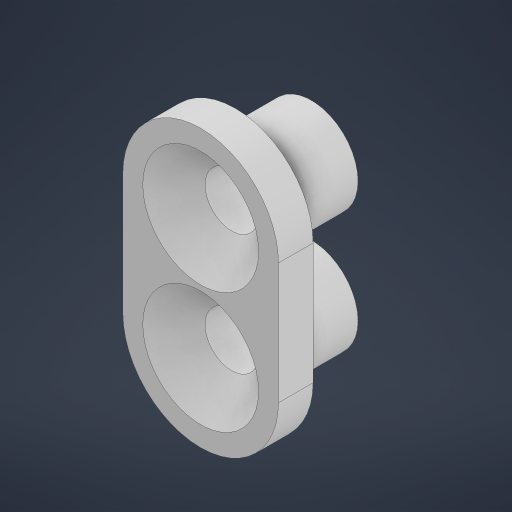
# Autodesk Inventor part: Stange halter
Saved by Autodesk Inventor 2024.2 (Build 282272000, 272)
## iProperties
Created: 2024-02-24
Part Number: Stange halter
Material: Generisch
Document SubType Name: Modeling
Designer: jacob
Density: 1 g/cm^3
Appearance: Vorgabe
Author: jacob
Autodesk Inventor part; units mm, degrees
ref_plane "YZ Plane" through (0, 0, 0) normal (1, 0, 0) x (0, 1, 0)
ref_plane "XZ Plane" through (0, 0, 0) normal (0, 1, 0) x (-1, 0, 0)
ref_plane "XY Plane" through (0, 0, 0) normal (0, 0, 1) x (1, 0, 0)
sketch "Skizze1" plane through (0, 0, 0) normal (0, 0, 1) x (1, 0, 0)
  circle A0 centre (0, 0) radius 2.7
  circle A1 centre (0, -7) radius 2.7
  dimension "d22" = 5.4
  dimension "d23" = 7
  constraints: 2 centre point, 1 coincident, 1 equal radius, 1 vertical alignment
  measures "d22" diameter of A0
  measures "d23" distance of point (0, 0) A1.centre
extrude "Extrusion1" add sketch "Skizze1" along normal blind 5.2
sketch "Skizze2" plane through (0, 0, 5.2) normal (0, 0, 1) x (1, 0, 0)
  arc A0 (-3, -7) -> (3, -7) centre (0, -7) ccw projected
  arc A1 (-3, -7) -> (3, -7) centre (0, -7) ccw projected
  line L0 (-3, 0) -> (-3, -7)
  arc A2 (3, 0) -> (-3, 0) centre (0, 0) ccw
  line L1 (3, -7) -> (3, 0)
  arc A3 (-3, -7) -> (3, -7) centre (0, -7) ccw
  line L2 (-3, 0) -> (-3, -7) projected
  arc A4 (-3, -7) -> (3, -7) centre (0, -7) ccw projected
  line L3 (3, -7) -> (3, 0) projected
  arc A5 (3, 0) -> (-3, 0) centre (0, 0) ccw projected
  line L4 (-3, 0) -> (-3, -7) projected
  line L5 (-3, 0) -> (-3, -7) projected
  arc A6 (-3, -7) -> (3, -7) centre (0, -7) ccw projected
  arc A7 (-3, -7) -> (3, -7) centre (0, -7) ccw projected
  line L6 (3, -7) -> (3, 0) projected
  line L7 (3, -7) -> (3, 0) projected
  arc A8 (3, 0) -> (-3, 0) centre (0, 0) ccw projected
  arc A9 (3, 0) -> (-3, 0) centre (0, 0) ccw projected
  line L8 (-4.5, 0) -> (-4.5, -7)
  arc A10 (-4.5, -7) -> (4.5, -7) centre (0, -7) ccw
  line L9 (4.5, -7) -> (4.5, 0)
  arc A11 (4.5, 0) -> (-4.5, 0) centre (0, 0) ccw
  dimension "d4" = 9
  constraints: 6 end point, 4 centre point, 4 point on circle, 4 tangent, 3 coincident, 1 parallel, 1 vertical
  measures "d4" distance between parallel lines of L8 L9
extrude "Extrusion2" add sketch "Skizze2" along normal blind 2 contours L0 A2 L1 A0 | A11 L9 A10 L8
sketch "Skizze3" plane through (0, 0, 7.2) normal (0, 0, 1) x (1, 0, 0)
  point P0 (0, 0)
  point P1 (0, 0)
  point P2 (0, -7)
  dimension "d7" = 7
  constraints: 1 coincident, 1 vertical alignment
  measures "d7" distance of point (0, 0) point (0, -7)
hole "Bohrung1" at (0, 0, 7.2) at (0, -7, 7.2) direction (0, 0, -1) diameter 3.1 end through all
chamfer "Fasen1" distance 2.8 angle 45 2 edges at (0, 1.55, 7.2) (0, -5.45, 7.2)
sketch "Skizze5" plane through (0, 0, 5.2) normal (0, 0, -1) x (-1, 0, 0)
  circle A0 centre (0, -7) radius 2.7 projected
  line L0 (4.5, 0) -> (4.5, -7) projected
  arc A1 (-4.5, -7) -> (4.5, -7) centre (0, -7) ccw projected
  line L1 (-4.5, -7) -> (-4.5, 0) projected
  arc A2 (4.5, 0) -> (-4.5, 0) centre (0, 0) ccw projected
  circle A3 centre (0, 0) radius 2.7 projected
  circle A4 centre (0, -7) radius 2.35 projected
  circle A5 centre (0, 0) radius 2.35 projected
extrude "Extrusion4" add sketch "Skizze5" along normal blind 1 contours L0 A1 L1 A2
sketch "Skizze6" plane through (0, 0, 7.2) normal (0, 0, 1) x (1, 0, 0)
  arc A0 (-2.5831, -3.5) -> (2.5831, -3.5) centre (0, -7) ccw projected
  arc A1 (2.5831, -3.5) -> (-2.5831, -3.5) centre (0, 0) ccw projected
  arc A2 (-4.5, -7) -> (4.5, -7) centre (0, -7) ccw projected
  line L0 (-4.5, -7) -> (-4.5, 0) projected
  arc A3 (4.5, 0) -> (-4.5, 0) centre (0, 0) ccw projected
  line L1 (4.5, 0) -> (4.5, -7) projected
extrude "Extrusion5" cut sketch "Skizze6" against normal blind 1 contours A1 A0 | L0 A3 L1 A2
sketch "Skizze7" plane through (0, 0, 0) normal (0, 0, -1) x (-1, 0, 0)
  circle A0 centre (0, 0) radius 1.55 projected
  circle A1 centre (0, 0) radius 2.7 projected
  circle A2 centre (0, -7) radius 1.55 projected
  circle A3 centre (0, -7) radius 2.7 projected
extrude "Extrusion6" add sketch "Skizze7" along normal blind 0.2
